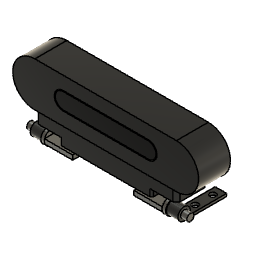
深度相机 v2 (Autodesk Fusion 360 design; units mm, degrees)
Autodesk Fusion 360 part; units mm, degrees
sketch "草图1" plane through (0, 0, 0) normal (0, 1, 0) x (1, 0, 0)
  line L0 (40, -12.5) -> (-40, -12.5)
  line L1 (-40, -12.5) -> (-40, 12.5)
  line L2 (-40, 12.5) -> (40, 12.5)
  line L3 (40, 12.5) -> (40, -12.5)
  line L4 (40, -12.5) -> (-40, 12.5) construction
  line L5 (-40, -12.5) -> (40, 12.5) construction
  arc A0 (-40, 12.5) -> (-40, -12.5) centre (-40, 0) ccw
  arc A1 (40, -12.5) -> (40, 12.5) centre (40, 0) ccw
  dimension "d1" = 25
  dimension "d2" = 80
  constraint horizontal L0
  constraint perpendicular L0 L1
  constraint parallel L0 L2
  constraint parallel L1 L3
  constraint coincident L4 origin
  constraint coincident L5 origin
  constraint coincident L1 L2.start
  constraint midpoint L1 A0.centre
  constraint midpoint L3 A1.centre
  measures "d1" distance of L0.end L1.end
  measures "d2" distance of L1.end L2.end
extrude "拉伸1" add sketch "草图1" along normal blind 18 makes body 1
sketch "草图2" plane through (0, 0, 0) normal (0, -1, 0) x (1, 0, 0)
  arc A0 (-40, 12.5) -> (-40, -12.5) centre (-40, 0) ccw
  line L0 (-40, -12.5) -> (40, -12.5)
  arc A1 (40, -12.5) -> (40, 12.5) centre (40, 0) ccw
  line L1 (40, 12.5) -> (-40, 12.5)
  line L2 (24, -5) -> (-24, -5)
  line L3 (-24, -5) -> (-24, 5)
  line L4 (-24, 5) -> (24, 5)
  line L5 (24, 5) -> (24, -5)
  line L6 (24, -5) -> (-24, 5) construction
  line L7 (-24, -5) -> (24, 5) construction
  arc A2 (-24, 5) -> (-24, -5) centre (-24, 0) ccw
  arc A3 (24, -5) -> (24, 5) centre (24, 0) ccw
  dimension "d5" = 10
  dimension "d6" = 48
  constraint horizontal L2
  constraint perpendicular L2 L3
  constraint parallel L2 L4
  constraint parallel L3 L5
  constraint coincident L6 origin
  constraint coincident L7 origin
  constraint midpoint L3 A2.centre
  constraint midpoint L5 A3.centre
  measures "d5" distance of L2.end L3.end
  measures "d6" distance of L2.start L2.end
extrude "拉伸2" cut sketch "草图2" against normal blind 5 contours L2 L3 L4 L5 | L5 A3 | L3 A2 bodies 1
sketch "草图3" plane through (0, 5, 0) normal (0, -1, 0) x (1, 0, 0)
  arc A0 (-24, 5) -> (-24, -5) centre (-24, 0) ccw
  line L0 (-24, -5) -> (24, -5)
  arc A1 (24, -5) -> (24, 5) centre (24, 0) ccw
  line L1 (24, 5) -> (-24, 5)
  line L2 (-24, -4.5) -> (24, -4.5)
  arc A2 (24, -4.5) -> (24, 4.5) centre (24, 0) ccw
  line L3 (24, 4.5) -> (-24, 4.5)
  arc A3 (-24, 4.5) -> (-24, -4.5) centre (-24, 0) ccw
  dimension "d9" = -0.5
extrude "拉伸3" add sketch "草图3" along normal blind 5 separate body contours L2 A2 L3 A3 makes body 2
sketch "草图4" plane through (0, 0, -12.5) normal (0, 0, -1) x (1, 0, 0)
  line L0 (40, 0) -> (-40, 0)
  line L1 (-40, 0) -> (-40, -18)
  line L2 (-40, -18) -> (40, -18)
  line L3 (40, -18) -> (40, 0)
  line L4 (0, 20) -> (0, -38.0009)
  line L5 (-38, 0) -> (-20, 0)
  line L6 (-20, 0) -> (-20, -16)
  line L7 (-22, -18) -> (-38, -18)
  line L8 (-40, -16) -> (-40, -2)
  line L9 (-38, -18) -> (-40, -16)
  line L10 (-20, -16) -> (-22, -18)
  line L11 (-38, 0) -> (-40, -2)
  line L12 (38, 0) -> (20, 0)
  line L13 (38, 0) -> (40, -2)
  line L14 (40, -16) -> (40, -2)
  line L15 (20, 0) -> (20, -16)
  line L16 (20, -16) -> (22, -18)
  line L17 (22, -18) -> (38, -18)
  line L18 (38, -18) -> (40, -16)
  line L19 (-20, 0) -> (20, 0)
  line L20 (20, 0) -> (20, -5)
  line L21 (20, -5) -> (-20, -5)
  line L22 (-20, -5) -> (-20, 0)
  point P0 (-40, 0)
  point P1 (-20, -18)
  point P2 (-40, -18)
  dimension "d12" = 2
  dimension "d13" = 2
  dimension "d14" = 2
  dimension "d15" = 2
  dimension "d16" = 2
  dimension "d17" = 2
  dimension "d18" = 40
  dimension "d19" = 16
  dimension "d20" = 5
  constraint vertical L4
  constraint horizontal L5
  constraint vertical L6
  constraint horizontal L7
  constraint vertical L8
  constraint coincident L2 P1
  constraint coincident L0 P0
  constraint coincident P2 L7
  constraint coincident P2 L8
  constraint coincident P1 L6
  constraint coincident P1 L7
  constraint coincident P0 L5
  constraint coincident P0 L8
  constraint symmetric L4 L5.end L12.end
  constraint symmetric L4 L7.end L17.end
  constraint symmetric L4 L8.start L14.start
  constraint symmetric L4 L6.end L15.end
  constraint symmetric L4 L7.start L16.end
  constraint symmetric L4 L5.start L12.start
  constraint symmetric L4 L8.end L13.end
  constraint coincident origin L4
  constraint horizontal L19
  constraint vertical L20
  constraint horizontal L21
  constraint vertical L22
  constraint coincident L15 L20.end
  measures "d12" distance of P2 L7.end
  measures "d13" distance of P2 L8.start
  measures "d14" distance of P1 L6.end
  measures "d15" distance of P1 L7.start
  measures "d16" distance of P0 L5.start
  measures "d17" distance of P0 L8.end
  measures "d18" distance of L6 L15
  measures "d19" distance of L7.end L7.start
  measures "d20" distance of L5.end L21.end
extrude "拉伸4" add sketch "草图4" along normal blind 6 separate body contours L0 L2 L3 L12 L13 L14 L15 L16 L17 L18 L20 | L0 L4 L15 L19 L20 L21 | L0 L4 L6 L19 L21 L22 | L0 L1 L2 L5 L6 L7 L8 L9 L10 L11 L22 makes body 3
sketch "草图5" plane through (0, 0, -18.5) normal (0, 0, -1) x (1, 0, 0)
  line L0 (20, -16) -> (22, -18)
  line L1 (22, -18) -> (38, -18)
  line L2 (38, -18) -> (40, -16)
  line L3 (40, -16) -> (40, -2)
  line L4 (40, -2) -> (38, 0)
  line L5 (38, 0) -> (-38, 0)
  line L6 (-38, 0) -> (-40, -2)
  line L7 (-40, -2) -> (-40, -16)
  line L8 (-40, -16) -> (-38, -18)
  line L9 (-38, -18) -> (-22, -18)
  line L10 (-22, -18) -> (-20, -16)
  line L11 (-20, -16) -> (-20, -5)
  line L12 (-20, -5) -> (20, -5)
  line L13 (20, -5) -> (20, -16)
  line L14 (0, 7) -> (0, -30)
  line L15 (-25, 0) -> (-20, 0)
  line L16 (-20, 0) -> (-20, -4)
  line L17 (-21, -5) -> (-25, -5)
  line L18 (-26, -4) -> (-26, -1)
  line L19 (-25, 0) -> (-26, -1)
  line L20 (-25, -5) -> (-26, -4)
  line L21 (-20, -4) -> (-21, -5)
  line L22 (25, 0) -> (20, 0)
  line L23 (25, 0) -> (26, -1)
  line L24 (26, -4) -> (26, -1)
  line L25 (25, -5) -> (26, -4)
  line L26 (21, -5) -> (25, -5)
  line L27 (20, -4) -> (21, -5)
  line L28 (20, 0) -> (20, -4)
  line L29 (-20, 0) -> (20, 0)
  line L30 (20, 0) -> (20, -4)
  line L31 (20, -4) -> (-20, -4)
  line L32 (-20, -4) -> (-20, 0)
  point P0 (-26, 0)
  point P1 (-20, -5)
  point P2 (-26, -5)
  dimension "d23" = 1
  dimension "d24" = 1
  dimension "d25" = 1
  dimension "d26" = 1
  dimension "d27" = 1
  dimension "d28" = 1
  dimension "d29" = 52
  dimension "d30" = 4
  constraint perpendicular L5 L14
  constraint horizontal L15
  constraint vertical L16
  constraint horizontal L17
  constraint vertical L18
  constraint coincident L12 P1
  constraint coincident L5 P0
  constraint coincident P0 L15
  constraint coincident P0 L18
  constraint coincident P2 L17
  constraint coincident P2 L18
  constraint coincident P1 L16
  constraint coincident P1 L17
  constraint symmetric L14 L15.end L22.end
  constraint symmetric L14 L15.start L22.start
  constraint symmetric L14 L18.end L23.end
  constraint symmetric L14 L17.end L25.start
  constraint symmetric L14 L18.start L24.start
  constraint symmetric L14 L16.end L27.start
  constraint symmetric L14 L17.start L26.start
  constraint coincident origin L14
  constraint horizontal L29
  constraint vertical L30
  constraint horizontal L31
  constraint vertical L32
  measures "d23" distance of P0 L15.start
  measures "d24" distance of P0 L18.end
  measures "d25" distance of P2 L17.end
  measures "d26" distance of P2 L18.start
  measures "d27" distance of P1 L16.end
  measures "d28" distance of P1 L17.start
  measures "d29" distance of L18 L24
  measures "d30" distance of L17.end L17.start
extrude "拉伸5" add sketch "草图5" along normal blind 4 contours L5 L14 L16 L29 L31 L32 | L5 L14 L28 L29 L30 L31 | L5 L22 L23 L24 L25 L26 L27 L28 L30 | L5 L15 L16 L17 L18 L19 L20 L21 L32 bodies 3
sketch "草图6" plane through (0, 0, -12.5) normal (0, 0, -1) x (1, 0, 0)
  line L0 (40, 0) -> (-40, 0)
  line L1 (-40, 0) -> (-40, -18)
  line L2 (-40, -18) -> (40, -18)
  line L3 (40, -18) -> (40, 0)
  line L4 (-6, -12) -> (-14, -12)
  line L5 (-14, -12) -> (-14, -9)
  line L6 (-14, -9) -> (-6, -9)
  line L7 (-6, -9) -> (-6, -12)
  line L8 (-20, -16) -> (-20, -5)
  dimension "d33" = 3
  dimension "d34" = 8
  dimension "d35" = 6
  dimension "d36" = 6
  constraint horizontal L4
  constraint vertical L5
  constraint horizontal L6
  constraint vertical L7
  measures "d33" distance of L4.start L6.end
  measures "d34" distance of L4.start L4.end
  measures "d35" distance of L2 L4
  measures "d36" distance of L5 L8
extrude "拉伸6" cut sketch "草图6" against normal blind 4 contours L4 L5 L6 L7 bodies 1
sketch "草图7" plane through (0, 0, -22.5) normal (0, 0, -1) x (1, 0, 0)
  line L0 (21, -5) -> (25, -5)
  line L1 (25, -5) -> (26, -4)
  line L2 (26, -4) -> (26, -1)
  line L3 (26, -1) -> (25, 0)
  line L4 (25, 0) -> (-25, 0)
  line L5 (-25, 0) -> (-26, -1)
  line L6 (-26, -1) -> (-26, -4)
  line L7 (-26, -4) -> (-25, -5)
  line L8 (-25, -5) -> (-21, -5)
  line L9 (-21, -5) -> (-20, -4)
  line L10 (-20, -4) -> (20, -4)
  line L11 (20, -4) -> (21, -5)
  circle A0 centre (21.25, -2.6201) radius 1.75
  line L12 (0, -19) -> (0, 10)
  circle A1 centre (-21.25, -2.6201) radius 1.75
  dimension "d39" = 3.5
  dimension "d40" = 42.5
  constraint vertical L12
  constraint symmetric A0 L12 A1
  measures "d39" diameter of A0
extrude "拉伸7" cut sketch "草图7" against normal blind 4 contours A0 | A1 bodies 3
copy_body "实体->零部件1" bodies 1 removing the originals makes body 4 in component "Component'"
copy_body "实体->零部件2" bodies 2 removing the originals makes body 5 in component "Component''"
copy_body "实体->零部件3" bodies 3 removing the originals makes body 6 in component "Component'''"
sketch "草图8" plane through (0, 0, 0) normal (0, 1, 0) x (1, 0, 0)
  line L0 (23, -10) -> (7, -10)
  line L1 (7, -10) -> (7, -18)
  line L2 (7, -18) -> (23, -18)
  line L3 (23, -18) -> (23, -10)
  circle A0 centre (11, -14) radius 1.75
  dimension "d43" = 8
  dimension "d44" = 16
  dimension "d45" = 3.5
  dimension "d46" = 4
  dimension "d47" = 4
  constraint horizontal L0
  constraint vertical L1
  constraint horizontal L2
  constraint vertical L3
  measures "d43" distance of L0.start L2.end
  measures "d44" distance of L0.start L0.end
  measures "d45" diameter of A0
  measures "d46" distance of L1 A0.centre
  measures "d47" distance of L0 A0.centre
extrude "拉伸8" add sketch "草图8" along normal blind 2.5 separate body makes body 7
sketch "草图9" plane through (23, 0, 0) normal (1, 0, 0) x (0, 1, 0)
  line L0 (0, 18) -> (0, 10)
  line L1 (0, 10) -> (2.5, 10)
  line L2 (2.5, 10) -> (2.5, 18)
  line L3 (2.5, 18) -> (0, 18)
  circle A0 centre (1.25, 14) radius 4
  dimension "d50" = 8
  dimension "d51" = 1.25
  measures "d50" diameter of A0
  measures "d51" distance of L0 A0.centre
extrude "拉伸9" add sketch "草图9" along normal blind 2 contours L0 L2 A0 | L0 A0 | L2 A0 bodies 7
sketch "草图10" plane through (25, 0, 0) normal (1, 0, 0) x (0, 1, 0)
  circle A0 centre (1.25, 14) radius 4
  circle A1 centre (1.25, 14) radius 2
  dimension "d54" = 4
  constraint concentric A0 A1
  measures "d54" diameter of A1
extrude "拉伸10" add sketch "草图10" along normal blind 10 contours A1 bodies 7
copy_body "实体->零部件4" bodies 7 removing the originals makes body 8 in component "Component''''"
sketch "草图11" plane through (0, 0, 0) normal (0, 1, 0) x (1, 0, 0)
  line L0 (25.6264, 17.022) -> (1.6264, 17.022)
  line L1 (1.6264, 17.022) -> (1.6264, 15.522)
  line L2 (1.6264, 15.522) -> (25.6264, 15.522)
  line L3 (25.6264, 15.522) -> (25.6264, 17.022)
  circle A0 centre (25.6264, 19.022) radius 3.5
  circle A1 centre (25.6264, 19.022) radius 2
  dimension "d57" = 7
  dimension "d58" = 1.5
  dimension "d59" = 24
  dimension "d60" = 4
  constraint horizontal L0
  constraint vertical L1
  constraint horizontal L2
  constraint vertical L3
  constraint tangent L2 A0
  constraint coincident L3 A0.centre
  constraint concentric A0 A1
  measures "d57" diameter of A0
  measures "d58" distance of L0.start L2.end
  measures "d59" distance of L1.end L2.end
  measures "d60" diameter of A1
extrude "拉伸11" add sketch "草图11" along normal blind 6.5 separate body makes body 9
sketch "草图12" plane through (0, 0, -15.522) normal (0, 0, 1) x (-1, 0, 0)
  line L0 (-1.6264, 0) -> (-25.6264, 0)
  line L1 (-25.6264, 0) -> (-25.6264, -6.5)
  line L2 (-25.6264, -6.5) -> (-1.6264, -6.5)
  line L3 (-1.6264, -6.5) -> (-1.6264, 0)
  circle A0 centre (-16.1264, -3.25) radius 1.75
  circle A1 centre (-6.1264, -3.25) radius 1.75
  dimension "d63" = 3.5
  dimension "d64" = 3.5
  dimension "d65" = 3.25
  dimension "d66" = 3.25
  dimension "d67" = 4.5
  dimension "d68" = 14.5
  measures "d63" diameter of A0
  measures "d64" diameter of A1
  measures "d65" distance of L2 A0.centre
  measures "d66" distance of L2 A1.centre
  measures "d67" distance of L3 A1.centre
  measures "d68" distance of L3 A0.centre
extrude "拉伸12" cut sketch "草图12" against normal blind 1.5 contours A0 | A1 bodies 9
copy_body "实体->零部件5" bodies 9 removing the originals makes body 10 in component "Component'''''"
component "Component'" placed x (1, 0, 0) y (0, 1, 0) z (0, 0, 1) at (-10.7085, -3.6184, -2.5938)
component "Component''" placed x (1, 0, 0) y (0, 1, 0) z (0, 0, 1) at (-10.7085, -3.6184, -2.5938)
component "Component'''" placed x (1, 0, 0) y (0, 1, 0) z (0, 0, 1) at (-10.7085, -3.6184, -2.5938)
component "Component''''" placed x (1, 0, 0) y (0, 0, -1) z (0, 1, 0) at (-0.4585, -14.9983, -25.0938)
component "Component'''''" placed x (0, -0.996195, -0.087156) y (-1, 0, 0) z (0, 0.087156, -0.996195) at (31.0415, 26.1884, -43.06)
component "Component''''" placed x (-1, 0, 0) y (0, 0, 1) z (0, 1, 0) at (-20.9585, -14.9983, -27.5938)
component "Component'''''" placed x (0, -1, 0) y (-1, 0, 0) z (0, 0, -1) at (-45.9585, 24.6281, -45.3659)
equation "d13 = d12"
equation "d15 = d14"
equation "d17 = d16"
equation "d24 = d23"
equation "d26 = d25"
equation "d28 = d27"
